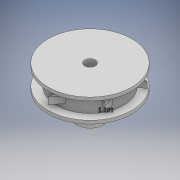
# Autodesk Inventor part: intermediateSpindle
Saved by Autodesk Inventor 2018 (Build 220112000, 112)
## iProperties
Created: 2017-10-22
Part Number: intermediateSpindle
Material: Generic
Document SubType Name: Modeling
Designer: Prakash
Density: 1 g/cm^3
Appearance: Default
Author: Prakash
Autodesk Inventor part; units mm, degrees
note: some values were not read from the file. Chosen so that the rebuilt part matches the saved one: direction of "Hole2".
ref_plane "XZ Plane" through (0, 0, 0) normal (0, 1, 0) x (-1, 0, 0)
sketch "Sketch1" plane through (0, 0, 0) normal (0, 0, 1) x (1, 0, 0)
  circle A0 centre (0, 0) radius 20
  circle A1 centre (0, 0) radius 25
  circle A2 centre (0, 0) radius 3.175
  circle A3 centre (0, 0) radius 8.175
  dimension "d18" = 6.35
  dimension "d19" = 16.35
  dimension "d40" = 40
  dimension "d41" = 5
  constraints: 4 centre point, 4 coincident
  measures "d18" diameter of A2
  measures "d19" diameter of A3
  measures "d40" diameter of A0
  measures "d41" radial gap between concentric circles of A1 A0
extrude "Extrusion1" add sketch "Sketch1" along normal blind 14 contours A0 | A2 | A3
extrude "Extrusion2" add sketch "Sketch1" along normal blind 2 contours A1
sketch "Sketch2" plane through (0, 0, 14) normal (0, 0, 1) x (1, 0, 0)
  circle A0 centre (0, 0) radius 20 projected
  circle A1 centre (0, 0) radius 25 projected
extrude "Extrusion3" add sketch "Sketch2" against normal blind 2
ref_plane "Work Plane1" through (0, 0, 7) normal (0, 0, -1) x (-1, 0, 0)
extrude "Extrusion5" cut sketch "Sketch1" along normal up to surface (14 mm away) contours A2
extrude "Extrusion6" add sketch "Sketch1" against normal blind 14 contours A3
ref_plane "Work Plane2" through (8.175, 0, 0) normal (1, 0, 0) x (0, 1, 0)
sketch "Sketch9" plane through (0, 0, 7) normal (0, 0, -1) x (-1, 0, 0)
  circle A0 centre (0, 0) radius 20 projected
  line L0 (0, -20) -> (0, -25) construction
  circle A1 centre (0, 0) radius 25 projected
  arc A2 (0, -20) -> (0, -25) centre (7.5993, -22.5) ccw
  line L1 (0, -25) -> (-4.6567, -19.4503)
  circle A3 centre (0, 0) radius 20
  line L2 (17.3205, -10) -> (21.6506, -12.5) construction
  line L3 (21.6506, -12.5) -> (14.5161, -13.758)
  arc A4 (17.3205, -10) -> (21.6506, -12.5) centre (23.2852, -4.6688) ccw
  line L4 (17.3205, 10) -> (21.6506, 12.5) construction
  line L5 (21.6506, 12.5) -> (19.1728, 5.6923)
  arc A5 (17.3205, 10) -> (21.6506, 12.5) centre (15.6859, 17.8312) ccw
  line L6 (0, 20) -> (0, 25) construction
  line L7 (0, 25) -> (4.6567, 19.4503)
  arc A6 (0, 20) -> (0, 25) centre (-7.5993, 22.5) ccw
  line L8 (-17.3205, 10) -> (-21.6506, 12.5) construction
  line L9 (-21.6506, 12.5) -> (-14.5161, 13.758)
  arc A7 (-17.3205, 10) -> (-21.6506, 12.5) centre (-23.2852, 4.6688) ccw
  line L10 (-17.3205, -10) -> (-21.6506, -12.5) construction
  line L11 (-21.6506, -12.5) -> (-19.1728, -5.6923)
  arc A8 (-17.3205, -10) -> (-21.6506, -12.5) centre (-15.6859, -17.8312) ccw
  point P0 (0, -22.5)
  point P1 (19.4856, -11.25)
  point P2 (19.4856, 11.25)
  point P3 (0, 22.5)
  point P4 (-19.4856, 11.25)
  point P5 (-19.4856, -11.25)
  dimension "d58" = 8
  dimension "d59" = 40
  dimension "d62" = 360
  constraints: 24 end point, 12 point on circle, 7 centre point, 2 vertical, 1 coincident, 1 midpoint, 1 vertical alignment, 64 other
  measures "d58" radius of A2
  measures "d59" angle of L1 L0
extrude "Extrusion9" add sketch "Sketch9" along normal mid plane 4 contours A0 A5 L5 | A4 L3 A0 | A0 A6 L7 | A2 L1 A0 | L9 A0 A7 | L11 A0 A8
sketch "Sketch10" plane through (8.175, 0, 0) normal (1, 0, 0) x (0, 1, 0)
  line L0 (0, 0) -> (0, -14) construction
  line L1 (-8.175, -14) -> (8.175, -14) construction
  circle A0 centre (0, -7) radius 2.6543
  circle A1 centre (0, -7) radius 2.5273
  dimension "d66" = 5.3086
  dimension "d67" = 5.0546
  constraints: 2 centre point, 2 end point, 2 midpoint, 1 coincident
  measures "d66" diameter of A0
  measures "d67" diameter of A1
extrude "Extrusion10" cut sketch "Sketch10" against normal blind 3.81 contours A1
loft "Loft1" cut profiles "Sketch10" section 2 edges at (4.365, -2.5273, -7) contours A0 | A1
hole "Hole2" at (8.175, 0, -7) direction (-1, 0, 0) diameter 3.797 end up to surface clearance for "Flat Head Machine Screw (82)" size "#6" standard "Ansi Unified Screw Threads"
body "Solid1"
